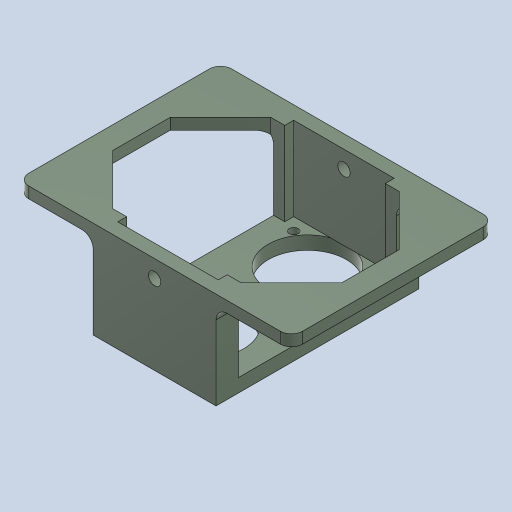
# Autodesk Inventor part: Ultrasonic_holderV4
Saved by Autodesk Inventor 2023 (Build 270158000, 158)
## iProperties
Created: 2022-06-24
Part Number: Ultrasonic_holderV4
Material: ABS プラスチック
Document SubType Name: Modeling
Designer: legot
Density: 1.06 g/cm^3
Appearance: 滑らか - 白
Mass: 4.73846 g
Surface Area: 51.1864 cm^2
Volume: 4.47025 cm^3
Author: legot
Autodesk Inventor part; units mm, degrees
ref_plane "YZ Plane" through (0, 0, 0) normal (1, 0, 0) x (0, 1, 0)
ref_plane "XZ Plane" through (0, 0, 0) normal (0, 1, 0) x (-1, 0, 0)
ref_plane "XY Plane" through (0, 0, 0) normal (0, 0, 1) x (1, 0, 0)
sketch "スケッチ1" plane through (0, 0, 0) normal (0, 1, 0) x (-1, 0, 0)
  line L0 (11, 15.75) -> (-11, 15.75)
  line L1 (-11, 15.75) -> (-11, 0)
  line L2 (-11, 0) -> (11, 0)
  line L3 (11, 0) -> (11, 15.75)
  line L4 (11, 0) -> (-11, 0) construction
  line L5 (-11, 0) -> (-11, -15.75) construction
  line L6 (-11, -15.75) -> (11, -15.75) construction
  line L7 (11, -15.75) -> (11, 0) construction
  circle A0 centre (0, 8.5) radius 7 construction
  point P0 (0, 0)
  point P1 (0, 0)
  point P2 (0, 0)
  point P3 (0, 15.75)
  dimension "d0" = 31.5
  dimension "d1" = 22
  dimension "d2" = 14
  dimension "d9" = 8.5
  constraints: 16 end point, 4 parallel, 2 horizontal, 2 midpoint, 2 perpendicular, 1 centre point, 1 coincident, 1 collinear, 1 vertical alignment
  measures "d0" distance between parallel lines of L0 L6
  measures "d1" distance of L0.start L0.end
  measures "d2" diameter of A0
  measures "d9" distance of point (0, 0) A0.centre
extrude "押し出し1" add sketch "スケッチ1" against normal blind 2.4
sketch "スケッチ2" plane through (-11, 0, 15.75) normal (0, 0, 1) x (1, 0, 0)
  line L0 (0, 0) -> (22, 0) projected
  line L1 (0, -2.4) -> (22, -2.4)
  line L2 (22, -2.4) -> (22, 12.9409)
  line L3 (22, 12.9409) -> (0, 12.9409)
  line L4 (0, 12.9409) -> (0, -2.4)
  line L5 (0, 0) -> (22, 0) projected
  line L6 (22, -2.4) -> (0, -2.4) projected
  line L7 (22, 0) -> (22, -2.4) projected
  line L8 (0, 0) -> (0, -2.4) projected
  line L9 (11, 11.8409) -> (-17.1108, -11.7468) construction
  line L10 (-17.7535, -10.9808) -> (10.3572, 12.607) construction
  line L11 (10.3572, 12.607) -> (11.6428, 11.0749) construction
  line L12 (11.6428, 11.0749) -> (-16.468, -12.5129) construction
  line L13 (-16.468, -12.5129) -> (-17.7535, -10.9808) construction
  line L14 (0, 0) -> (22, 0) construction
  line L15 (22, 0) -> (22, 1.6) construction
  line L16 (22, 1.6) -> (0, 1.6) construction
  line L17 (0, 1.6) -> (0, 0) construction
  line L18 (2.5, 1.6) -> (19.5, 1.6)
  line L19 (19.5, 1.6) -> (19.5, 0)
  line L20 (19.5, 0) -> (2.5, 0)
  line L21 (2.5, 0) -> (2.5, 1.6)
  line L22 (-2.9253, 2.767) -> (9.7144, 13.373)
  line L23 (9.7144, 13.373) -> (12.2856, 10.3088)
  line L24 (12.2856, 10.3088) -> (-0.3542, -0.2972)
  line L25 (-0.3542, -0.2972) -> (-2.9253, 2.767)
  line L26 (0, 0) -> (-2.8602, -2.4)
  line L27 (-2.8602, -2.4) -> (0, -2.4)
  point P0 (22, 0)
  point P1 (11, 0)
  point P2 (11, 1.6)
  point P3 (-1.6397, 1.2349)
  dimension "d14" = 2
  dimension "d15" = 40
  dimension "d16" = 1.6
  dimension "d62" = 17
  dimension "d64" = 15.3409
  dimension "d65" = 4
  dimension "d66" = 16.5
  dimension "d67" = 1.1
  constraints: 46 end point, 10 parallel, 7 midpoint, 5 perpendicular, 5 point on line, 4 horizontal, 1 collinear, 1 vertical alignment
  measures "d14" distance of L12.end L10.start
  measures "d15" angle of L9 L0
  measures "d16" distance of L16.end L5.start
  measures "d62" distance of L18.start L18.end
  measures "d64" distance between parallel lines of L3 L1
  measures "d65" distance of L22.end L23.end
  measures "d66" distance of L22.start L22.end
  measures "d67" distance from line of L3 L9.start
extrude "押し出し2" add sketch "スケッチ2" along normal blind 2.4 contours L24 L23 L3 L2 L0 L19 L18 L21 | L0 L2 L1 L4 | L4 L22 L3 L23 L24 | L21 L18 L19 L0 | L4 L3 L22
sketch "スケッチ3" plane through (0, 0, 0) normal (1, 0, 0) x (0, 1, 0)
  line L0 (12.9409, 15.75) -> (12.9409, 18.15) projected
  line L1 (14.9409, 18.15) -> (12.9409, 18.15)
  line L2 (12.9409, 18.15) -> (12.9409, 0)
  line L3 (12.9409, 0) -> (14.9409, 0)
  line L4 (14.9409, 0) -> (14.9409, 18.15)
  point P0 (0, 0)
  dimension "d10" = 2
  constraints: 8 end point, 2 parallel, 1 horizontal, 1 horizontal alignment, 1 perpendicular
  measures "d10" distance of L1.start L0.end
extrude "押し出し3" add sketch "スケッチ3" along normal mid plane 49
sketch "スケッチ5" plane through (0, -2.4, 0) normal (0, -1, 0) x (1, 0, 0)
  line L0 (-11, 0) -> (11, 0) projected
  circle A0 centre (0, 9.2) radius 7
  point P0 (0, 0)
  point P1 (0, 0)
  point P2 (0, 0)
  dimension "d29" = 14
  dimension "d30" = 9.2
  constraints: 2 midpoint, 1 centre point, 1 vertical alignment
  measures "d29" diameter of A0
  measures "d30" distance of A0.centre point (0, 0)
extrude "押し出し5" cut sketch "スケッチ5" against normal up to surface (2.4 mm away)
hole "穴1" at (0, 11.8409, 15.75) direction (0, 0, 1) diameter 2.2 end through all both
sketch "スケッチ6" plane through (0, -2.4, 0) normal (0, -1, 0) x (1, 0, 0)
  line L0 (11, 0) -> (11, 18.15) projected
  line L1 (-11, 0) -> (-11, 18.15) projected
  line L2 (11, 18.15) -> (9, 18.15)
  line L3 (9, 18.15) -> (9, 14.15)
  line L4 (9, 14.15) -> (11, 14.15)
  line L5 (11, 14.15) -> (11, 18.15)
  line L6 (-11, 18.15) -> (-9, 18.15)
  line L7 (-9, 18.15) -> (-9, 14.15)
  line L8 (-9, 14.15) -> (-11, 14.15)
  line L9 (-11, 14.15) -> (-11, 18.15)
  point P0 (0, 0)
  point P1 (-11, 14.15)
  dimension "d34" = 4
  dimension "d61" = 2
  constraints: 16 end point, 4 parallel, 2 horizontal, 2 perpendicular, 1 collinear, 1 point on line
  measures "d34" distance of L2.end L3.end
  measures "d61" distance of L3.end L4.end
extrude "補強" add sketch "スケッチ6" against normal up to surface (15.3409 mm away)
mirror "ミラー2" about plane through (0, 0, 0) normal (0, 0, 1) of "押し出し1", "押し出し2", "穴1", "押し出し3", "押し出し5", "補強"
sketch "スケッチ7" plane through (-24.5, 14.9409, 18.15) normal (0, 1, 0) x (1, 0, 0)
  line L0 (0, 0) -> (49, 0) projected
  line L1 (49, 0) -> (49, 36.3) projected
  line L2 (0, 36.3) -> (49, 36.3) projected
  line L3 (0, 0) -> (0, 36.3) projected
  line L4 (4, 32.3) -> (45, 32.3)
  line L5 (45, 32.3) -> (45, 4)
  line L6 (45, 4) -> (4, 4)
  line L7 (4, 4) -> (4, 32.3)
  point P0 (24.5, 18.15)
  dimension "d37" = 4
  constraints: 8 end point, 3 other
  measures "d37" distance between parallel lines of L3 L7
extrude "穴抜き" cut sketch "スケッチ7" against normal up to surface (2 mm away) contours L4 L5 L6 L7
chamfer "面取り1" distance 9 angle 45 4 edges at (-20.5, 13.9409, -14.15) (-20.5, 13.9409, 14.15) (20.5, 13.9409, 14.15) (20.5, 13.9409, -14.15)
fillet "フィレット1" radius 2 4 edges at (24.5, 13.9409, 18.15) (-24.5, 13.9409, 18.15) (24.5, 13.9409, -18.15) (-24.5, 13.9409, -18.15)
sketch "スケッチ10" plane through (0, -2.4, 0) normal (0, -1, 0) x (1, 0, 0)
  line L0 (6.75, 13.5) -> (-6.75, 13.5) construction
  line L1 (-6.75, 13.5) -> (-6.75, -13.5) construction
  line L2 (-6.75, -13.5) -> (6.75, -13.5) construction
  line L3 (6.75, -13.5) -> (6.75, 13.5) construction
  point P0 (0, 0)
  point P1 (0, 13.5)
  point P2 (6.75, 0)
  dimension "d51" = 13.5
  dimension "d52" = 27
  constraints: 8 end point, 4 coincident, 2 midpoint, 2 parallel, 1 horizontal, 1 horizontal alignment, 1 perpendicular, 1 vertical alignment
  measures "d51" distance of L0.start L0.end
  measures "d52" distance of L2.end L0.start
hole "穴2" at (6.75, -2.4, 13.5) at (-6.75, -2.4, 13.5) at (6.75, -2.4, -13.5) at (-6.75, -2.4, -13.5) direction (0, 1, 0) diameter 1.6 depth 2.4
sketch "スケッチ11" plane through (0, 0, 0) normal (0, 1, 0) x (1, 0, 0)
  line L0 (-9, 15.75) -> (-9, 14.15) projected
  line L1 (-9, 14.15) -> (-11, 14.15) projected
  line L2 (-11, 14.15) -> (-11, -14.15) projected
  line L3 (-11, -14.15) -> (-9, -14.15) projected
  line L4 (-9, -14.15) -> (-9, -15.75) projected
  line L5 (-9, -15.75) -> (-2.4693, -15.75) projected
  line L6 (2.4693, -15.75) -> (9, -15.75) projected
  line L7 (9, -15.75) -> (9, -14.15) projected
  line L8 (9, -14.15) -> (11, -14.15) projected
  line L9 (11, -14.15) -> (11, 14.15) projected
  line L10 (11, 14.15) -> (9, 14.15) projected
  line L11 (9, 14.15) -> (9, 15.75) projected
  line L12 (2.4693, 15.75) -> (9, 15.75) projected
  line L13 (-9, 15.75) -> (-2.4693, 15.75) projected
  line L14 (-9, 15.75) -> (-2.4693, 15.75) projected
  line L15 (-2.4693, 15.75) -> (2.4693, 15.75) projected
  line L16 (2.4693, 15.75) -> (9, 15.75) projected
  line L17 (9, 15.75) -> (0, 15.75) projected
  line L18 (1.1, 15.75) -> (-1.1, 15.75) projected
  line L19 (0, 15.75) -> (-9, 15.75) projected
  line L20 (0, -15.75) -> (-9, -15.75) projected
  line L21 (-1.1, -15.75) -> (1.1, -15.75) projected
  line L22 (9, -15.75) -> (0, -15.75) projected
  line L23 (2.4693, -15.75) -> (9, -15.75) projected
  line L24 (-2.4693, -15.75) -> (2.4693, -15.75) projected
  line L25 (-9, -15.75) -> (-2.4693, -15.75) projected
  point P0 (0, 0)
  point P1 (-2.4693, -15.75)
  point P2 (-2.4693, 15.75)
extrude "押し出し10" cut sketch "スケッチ11" along normal through all
fillet "フィレット2" radius 2 4 edges at (-11, 12.9409, -16.15) (-11, 12.9409, 16.15) (11, 12.9409, -16.15) (11, 12.9409, 16.15)
